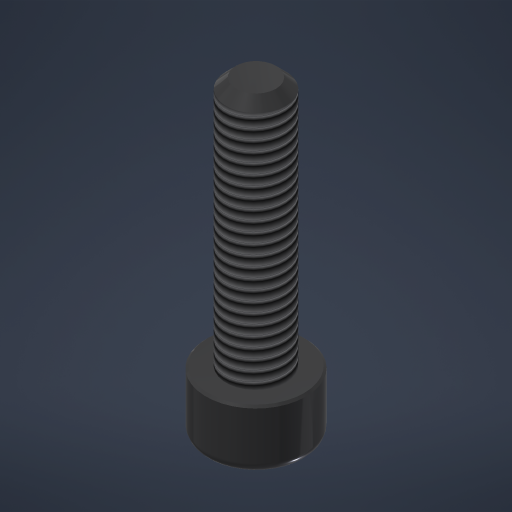
# Autodesk Inventor part: PERNO PARKER M6
Saved by Autodesk Inventor 2023 (Build 270158000, 158)
## iProperties
Created: 2006-10-30
Part Number: PERNO PARKER M6
Document SubType Name: Modeling
Designer: rbravo
Manufacturer: Standard
Standards Organization: Custom
Density: 1 g/cm^3
Material: Generic
Appearance: Dark Gray
Author: rbravo
Autodesk Inventor part; units mm, degrees
ref_plane "YZ Plane" through (0, 0, 0) normal (1, 0, 0) x (0, 1, 0)
ref_plane "XZ Plane" through (0, 0, 0) normal (0, 1, 0) x (-1, 0, 0)
ref_plane "XY Plane" through (0, 0, 0) normal (0, 0, 1) x (1, 0, 0)
sketch "Sketch1" plane through (0, 0, 0) normal (0, 0, 1) x (1, 0, 0)
  circle A0 centre (0, 0) radius 5
  dimension "d0" = 10
  constraints: 1 centre point
  measures "d0" diameter of A0
extrude "Extrusion1" add sketch "Sketch1" along normal blind 6
sketch "Sketch2" plane through (0, 0, 6) normal (0, 0, 1) x (1, 0, 0)
  circle A0 centre (0, 0) radius 5 projected
  circle A1 centre (0, 0) radius 3
  dimension "d3" = 6
  constraints: 1 centre point, 1 coincident
  measures "d3" diameter of A1
extrude "Extrusion2" add sketch "Sketch2" along normal blind 25 contours A1
thread "Thread1" size "M6x1" class "6g" standard "ANSI Metric M Profile" full length
chamfer "Chamfer1" distance 1 angle 45 1 edges at (-3, 0, 31)
chamfer "Chamfer2" distance 0.2 angle 45 1 edges at (-5, 0, 6)
fillet "Fillet1" radius 1 1 edges at (-5, 0, 0)
sketch "Sketch3" plane through (0, 0, 0) normal (0, 0, -1) x (-1, 0, 0)
  circle A0 centre (0, 0) radius 4 projected
  line L0 (1.5588, 2.4297) -> (2.8836, -0.135)
  line L1 (2.8836, -0.135) -> (1.3248, -2.5648)
  line L2 (1.3248, -2.5648) -> (-1.5588, -2.4297)
  line L3 (-1.5588, -2.4297) -> (-2.8836, 0.135)
  line L4 (-2.8836, 0.135) -> (-1.3248, 2.5648)
  line L5 (-1.3248, 2.5648) -> (1.5588, 2.4297)
  dimension "d15" = 5
  constraints: 12 end point, 1 coincident, 11 other
  measures "d15" distance between parallel lines of L5 L2
extrude "Extrusion3" cut sketch "Sketch3" against normal blind 5 contours L0 L1 L2 L3 L4 L5
body "Solid1"
